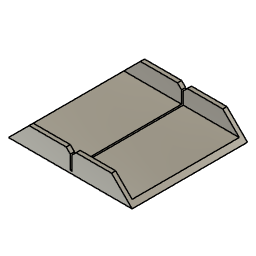
Wood Cut Template (Autodesk Fusion 360 design; units mm, degrees)
Autodesk Fusion 360 part; units mm, degrees
sketch "Sketch1" plane through (0, 0, 0) normal (0, 0, 1) x (1, 0, 0)
  line L0 (0, 0) -> (150, 0)
  line L1 (150, 0) -> (150, 140)
  line L2 (150, 140) -> (0, 140)
  line L3 (0, 140) -> (0, 0)
  dimension "d1" = 150
  dimension "d2" = 140
  constraint horizontal L0
  constraint vertical L1
  constraint horizontal L2
  constraint vertical L3
  constraint coincident L0.start L3.end
  measures "d1" distance of L0.start L0.end
  measures "d2" distance of L0.start L2.end
extrude "Extrude1" add sketch "Sketch1" along normal blind 5
sketch "Sketch2" plane through (0, 0, 5) normal (0, 0, 1) x (-1, 0, 0)
  line L0 (0, -140) -> (0, 0)
  line L1 (0, 0) -> (-150, 0)
  line L2 (-150, 0) -> (-150, -140)
  line L3 (-150, -140) -> (0, -140)
  line L4 (0, -140) -> (-150, -140)
  line L5 (-150, -140) -> (-150, -135)
  line L6 (-150, -135) -> (0, -135)
  line L7 (0, -135) -> (0, -140)
  line L8 (0, 0) -> (-150, 0)
  line L9 (-150, 0) -> (-150, -5)
  line L10 (-150, -5) -> (0, -5)
  line L11 (0, -5) -> (0, 0)
  line L12 (-75, -140) -> (-77, -140)
  line L13 (-77, -140) -> (-77, -135)
  line L14 (-77, -135) -> (-75, -135)
  line L15 (-75, -135) -> (-75, -140)
  line L16 (-75, 0) -> (-77, 0)
  line L17 (-77, 0) -> (-77, -5)
  line L18 (-77, -5) -> (-75, -5)
  line L19 (-75, -5) -> (-75, 0)
  dimension "d5" = 2
  dimension "d6" = 5
  dimension "d7" = 2
  dimension "d8" = 5
  constraint horizontal L4
  constraint vertical L5
  constraint horizontal L6
  constraint vertical L7
  constraint coincident L2 L5.end
  constraint coincident L0.start L3.end
  constraint horizontal L8
  constraint vertical L9
  constraint horizontal L10
  constraint vertical L11
  constraint coincident L2 L9.end
  constraint coincident L0.end L1.start
  constraint horizontal L12
  constraint vertical L13
  constraint horizontal L14
  constraint vertical L15
  constraint midpoint L4 L12.start
  constraint horizontal L16
  constraint vertical L17
  constraint horizontal L18
  constraint vertical L19
  constraint midpoint L8 L16.start
  measures "d5" distance of L12.start L12.end
  measures "d6" distance of L12.start L14.end
  measures "d7" distance of L16.start L16.end
  measures "d8" distance of L16.start L18.end
extrude "Extrude2" add sketch "Sketch2" along normal blind 20 contours L0 L3 L4 L6 L7 L15 | L0 L1 L8 L10 L11 L19 | L2 L3 L4 L5 L6 L13 | L1 L2 L8 L9 L10 L17
sketch "Sketch3" plane through (0, 0, 5) normal (0, 0, 1) x (-1, 0, 0)
  line L0 (-77, -5) -> (-150, -5)
  line L1 (-150, -5) -> (-150, -135)
  line L2 (-150, -135) -> (-77, -135)
  line L3 (-77, -135) -> (-77, -140)
  line L4 (-77, -140) -> (-75, -140)
  line L5 (-75, -140) -> (-75, -135)
  line L6 (-75, -135) -> (0, -135)
  line L7 (0, -135) -> (0, -5)
  line L8 (0, -5) -> (-75, -5)
  line L9 (-75, -5) -> (-75, 0)
  line L10 (-75, 0) -> (-77, 0)
  line L11 (-77, 0) -> (-77, -5)
  line L12 (-75, -140) -> (-77, -140)
  line L13 (-77, -140) -> (-77, 0)
  line L14 (-77, 0) -> (-75, 0)
  line L15 (-75, 0) -> (-75, -140)
  dimension "d11" = 2
  dimension "d12" = 140
  constraint horizontal L12
  constraint vertical L13
  constraint horizontal L14
  constraint vertical L15
  constraint coincident L4.end L5.start
  measures "d11" distance of L4.end L3.end
  measures "d12" distance of L4.end L9.end
extrude "Extrude3" cut sketch "Sketch3" against normal blind 2 contours L3 L4 L5 L9 L10 L11 L12 L13 L14 L15
chamfer "Chamfer1" distance 5 angle 45 4 edges at (75, 2.5, 25) (77, 2.5, 25) (75, 137.5, 25) (77, 137.5, 25)
chamfer "Chamfer2" distance 25 angle 45 4 edges at (150, 2.5, 25) (150, 137.5, 25) (0, 2.5, 25) (0, 137.5, 25)
